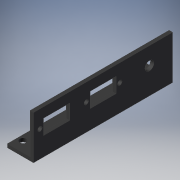
# Autodesk Inventor part: Pi-Output-Holder
Saved by Autodesk Inventor 2018 (Build 220112000, 112)
## iProperties
Created: 2018-09-21
Part Number: Pi-Output-Holder
Material: Generic
Document SubType Name: Modeling
Designer: bbramman
Density: 1 g/cm^3
Appearance: Default
Author: bbramman
Autodesk Inventor part; units mm, degrees
ref_plane "YZ Plane" through (0, 0, 0) normal (1, 0, 0) x (0, 1, 0)
ref_plane "XZ Plane" through (0, 0, 0) normal (0, 1, 0) x (-1, 0, 0)
ref_plane "XY Plane" through (0, 0, 0) normal (0, 0, 1) x (1, 0, 0)
sketch "Sketch2" plane through (0, 0, 0) normal (0, 1, 0) x (-1, 0, 0)
  line L0 (-9.525, 50.8) -> (9.525, 50.8)
  line L1 (9.525, 50.8) -> (9.525, -50.8)
  line L2 (9.525, -50.8) -> (-9.525, -50.8)
  line L3 (-9.525, -50.8) -> (-9.525, 50.8)
  line L4 (-9.525, 50.8) -> (9.525, -50.8) construction
  line L5 (9.525, 50.8) -> (-9.525, -50.8) construction
  line L6 (-9.525, 50.8) -> (5.715, 50.8)
  line L7 (5.715, 50.8) -> (5.715, 43.18)
  circle A0 centre (5.715, 43.18) radius 2.54
  line L8 (-9.525, -50.8) -> (5.715, -50.8)
  line L9 (5.715, -50.8) -> (5.715, -43.18)
  circle A1 centre (5.715, -43.18) radius 2.54
  point P0 (0, 0)
  dimension "d0" = 19.05
  dimension "d1" = 101.6
  dimension "d2" = 15.24
  dimension "d3" = 7.62
  dimension "d4" = 5.08
  dimension "d10" = 15.24
  dimension "d11" = 7.62
  dimension "d12" = 5.08
  constraints: 20 end point, 3 perpendicular, 2 centre point, 2 coincident, 2 midpoint, 2 parallel, 2 point on line, 1 horizontal
  measures "d0" distance of L1.end L2.end
  measures "d1" distance of L0.end L1.end
  measures "d2" distance of L0.start L6.end
  measures "d3" distance of L6.end L7.end
  measures "d4" diameter of A0
  measures "d10" distance of L2.end L8.end
  measures "d11" distance of L8.end L9.end
  measures "d12" diameter of A1
extrude "Extrusion3" add sketch "Sketch2" along normal blind 2.54
sketch "Sketch4" plane through (0, 2.54, 0) normal (0, 1, 0) x (1, 0, 0)
  line L0 (9.525, -50.8) -> (9.525, 50.8) projected
  line L1 (9.525, -50.8) -> (6.985, -50.8)
  line L2 (6.985, -50.8) -> (6.985, 50.8)
  line L3 (6.985, 50.8) -> (9.525, 50.8)
  line L4 (9.525, 50.8) -> (9.525, -50.8)
  point P0 (0, 0)
  dimension "d15" = 2.54
  dimension "d16" = 101.6
  constraints: 8 end point, 2 parallel, 1 horizontal, 1 perpendicular
  measures "d15" distance of L2.end L3.end
  measures "d16" distance of L1.end L2.end
extrude "Extrusion4" add sketch "Sketch4" along normal blind 29.21
sketch "Sketch5" plane through (9.525, 0, 50.8) normal (1, 0, 0) x (0, 0, -1)
  line L0 (0, 0) -> (101.6, 0) projected
  line L1 (101.6, 0) -> (101.6, 31.75) projected
  line L2 (0, 31.75) -> (101.6, 31.75) projected
  line L3 (0, 0) -> (0, 31.75) projected
  line L4 (0, 31.75) -> (101.6, 31.75) projected
  line L5 (0, 31.75) -> (33.8658, 31.75)
  line L6 (33.8658, 31.75) -> (67.724, 31.75)
  line L7 (16.9329, 31.75) -> (16.9329, 19.05)
  line L8 (50.7949, 31.75) -> (50.7949, 19.05)
  line L9 (67.724, 31.75) -> (101.6, 31.75)
  line L10 (84.662, 31.75) -> (84.662, 19.05)
  line L11 (16.9329, 19.05) -> (4.6829, 19.05)
  line L12 (4.6829, 19.05) -> (29.1829, 19.05)
  line L13 (50.7949, 19.05) -> (38.5449, 19.05)
  line L14 (38.5449, 19.05) -> (63.0449, 19.05)
  circle A0 centre (4.6829, 19.05) radius 1.651
  circle A1 centre (29.1829, 19.05) radius 1.651
  circle A2 centre (38.5449, 19.05) radius 1.651
  circle A3 centre (63.0449, 19.05) radius 1.651
  line L15 (7.4329, 13.55) -> (26.4329, 13.55)
  line L16 (26.4329, 13.55) -> (26.4329, 24.55)
  line L17 (26.4329, 24.55) -> (7.4329, 24.55)
  line L18 (7.4329, 24.55) -> (7.4329, 13.55)
  line L19 (7.4329, 13.55) -> (26.4329, 24.55) construction
  line L20 (26.4329, 13.55) -> (7.4329, 24.55) construction
  line L21 (41.2949, 13.55) -> (60.2949, 13.55)
  line L22 (60.2949, 13.55) -> (60.2949, 24.55)
  line L23 (60.2949, 24.55) -> (41.2949, 24.55)
  line L24 (41.2949, 24.55) -> (41.2949, 13.55)
  line L25 (41.2949, 13.55) -> (60.2949, 24.55) construction
  line L26 (60.2949, 13.55) -> (41.2949, 24.55) construction
  circle A4 centre (84.662, 19.05) radius 3.302
  point P0 (50.8, 0)
  dimension "d19" = 33.8658
  dimension "d20" = 33.8582
  dimension "d21" = 12.7
  dimension "d22" = 12.7
  dimension "d23" = 12.7
  dimension "d24" = 12.25
  dimension "d25" = 24.5
  dimension "d26" = 12.25
  dimension "d27" = 24.5
  dimension "d28" = 3.302
  dimension "d29" = 3.302
  dimension "d30" = 3.302
  dimension "d31" = 3.302
  dimension "d32" = 19
  dimension "d33" = 11
  dimension "d34" = 19
  dimension "d35" = 11
  dimension "d36" = 6.604
  constraints: 44 end point, 7 midpoint, 5 centre point, 5 coincident, 4 horizontal, 4 parallel, 4 point on line, 3 vertical, 2 perpendicular, 1 collinear
  measures "d19" distance of L2.start L5.end
  measures "d20" distance of L5.end L6.end
  measures "d21" distance of L7.start L7.end
  measures "d22" distance of L8.start L8.end
  measures "d23" distance of L10.start L10.end
  measures "d24" distance of L7.end L11.end
  measures "d25" distance of L11.end L12.end
  measures "d26" distance of L8.end L13.end
  measures "d27" distance of L13.end L14.end
  measures "d28" diameter of A0
  measures "d29" diameter of A1
  measures "d30" diameter of A2
  measures "d31" diameter of A3
  measures "d32" distance of L17.end L16.end
  measures "d33" distance of L16.end L15.end
  measures "d34" distance of L23.end L22.end
  measures "d35" distance of L22.end L21.end
  measures "d36" diameter of A4
extrude "Extrusion5" cut sketch "Sketch5" against normal through all contours A4 | A3 | A2 | L23 L22 L14 L8 | L8 L13 L24 L23 | A0 | L17 L16 L12 L7 | L7 L11 L18 L17 | L12 L16 L15 L18 L11 | L14 L22 L21 L24 L13
body "Solid1"
